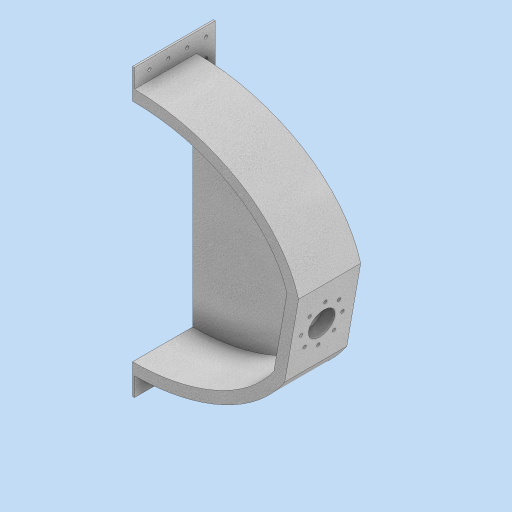
# Autodesk Inventor part: eggshellCorePrinted
Saved by Autodesk Inventor 2023 (Build 270158000, 158)
## iProperties
Created: 2026-03-19
Part Number: eggshellCorePrinted
Material: GFRC
Document SubType Name: Modeling
Designer: Nathann
Density: 1.7 g/cm^3
Appearance: Flat - Polished Gray
Mass: 7308.18 g
Surface Area: 8699.88 cm^2
Volume: 7308.18 cm^3
Author: Nathann
Autodesk Inventor part; units mm, degrees
ref_plane "YZ Plane" through (0, 0, 0) normal (1, 0, 0) x (0, 1, 0)
ref_plane "XZ Plane" through (0, 0, 0) normal (0, 1, 0) x (-1, 0, 0)
ref_plane "XY Plane" through (0, 0, 0) normal (0, 0, 1) x (1, 0, 0)
sketch "Sketch1" plane through (0, 0, 0) normal (0, 0, 1) x (1, 0, 0)
  ellipse E0 centre (0, 0) end of major axis (0, 330) minor radius 450 (0, -330) -> (0, 330) ccw
  ellipse E1 centre (0, 0) end of major axis (420, 0) minor radius 300 (0, -300) -> (0, 300) ccw
  line L0 (0, 300) -> (0, 330)
  line L1 (0, -300) -> (0, -330)
  line L2 (420, 0) -> (450, 0)
  dimension "d0" = 420
  dimension "d1" = 450
  dimension "d2" = 300
  dimension "d3" = 330
  constraints: 6 end point, 2 coincident, 2 point on line, 1 horizontal, 10 other
extrude "Extrusion1" add sketch "Sketch1" along normal blind 160
sketch "Sketch3" plane through (0, 0, 0) normal (0, 0, -1) x (-1, 0, 0)
  ellipse E0 centre (0, 0) end of major axis (420, 0) minor radius 300 (0, 300) -> (0, -300) ccw projected
  line L0 (-410.6033, 63.104) -> (-375.8737, -133.8576)
  line L1 (-375.8737, -133.8576) -> (-428.5073, -143.1383)
  line L2 (-428.5073, -143.1383) -> (-456.291, 14.4309)
  line L3 (0, 300) -> (0, -300) projected
  ellipse E1 centre (0, 0) end of major axis (450, 0) minor radius 330 (0, 330) -> (0, -330) ccw projected
  line L4 (-456.291, 14.4309) -> (-439.6592, 70.3382)
  line L5 (-428.5073, -143.1383) -> (-336.4493, -219.1451)
  line L6 (-336.4493, -219.1451) -> (-375.8737, -133.8576)
  line L7 (-410.6033, 63.104) -> (-439.6592, 70.3382)
  line L8 (-393.2385, -35.3768) -> (260.9914, 90.2506)
  line L9 (260.9914, 90.2506) -> (260.9914, 44.7879)
  line L10 (260.9914, 44.7879) -> (0, 40.1342)
  dimension "d8" = 200
  dimension "d9" = 10
  dimension "d12" = 45.4627
  dimension "d13" = 160
  constraints: 20 end point, 2 perpendicular, 2 point on line, 1 midpoint, 1 vertical, 9 other
  measures "d8" distance of L0.start L0.end
  measures "d9" angle of L3 L0
  measures "d12" distance of L8.end L9.end
  measures "d13" distance of L1.end L2.end
extrude "Extrusion2" add sketch "Sketch3" against normal blind 160 contours L0 E0
ref_plane "Work Plane2" through (0, 0, 0) normal (0, 0, -1) x (-1, 0, 0)
sketch "Sketch8" plane through (0, 0, 0) normal (0, 0, -1) x (-1, 0, 0)
  ellipse E0 centre (0, 0) end of major axis (450, 0) minor radius 330 (0, 330) -> (0, -330) ccw projected
  line L0 (0, -300) -> (0, -330) projected
  ellipse E1 centre (0, 0) end of major axis (420, 0) minor radius 300 (-375.8737, -133.8576) -> (0, -300) ccw projected
  line L1 (-375.8737, -133.8576) -> (-410.6033, 63.104) projected
  ellipse E2 centre (0, 0) end of major axis (420, 0) minor radius 300 (0, 300) -> (-410.6033, 63.104) ccw projected
  line L2 (0, 330) -> (0, 300) projected
  ellipse E3 centre (0, 0) end of major axis (420, 0) minor radius 300 (-375.8737, -133.8576) -> (0, -300) ccw projected
  line L3 (0, -300) -> (0, 300)
  point P0 (0, -300)
  constraints: 2 end point, 1 vertical, 5 other
extrude "Extrusion7" add sketch "Sketch8" along normal blind 5
ref_plane "Work Plane3" through (405.4179, -139.067, 0) normal (-0.9848078, 0.1736482, 0) x (0, 0, 1)
sketch "Sketch9" plane through (405.4179, -139.067, 0) normal (-0.9848078, 0.1736482, 0) x (0, 0, 1)
  line L0 (-87.5266, 298.4814) -> (215.3081, 298.4814)
  line L1 (215.3081, 298.4814) -> (215.3081, -153.555)
  line L2 (215.3081, -153.555) -> (-87.5266, -153.555)
  line L3 (-87.5266, -153.555) -> (-87.5266, 298.4814)
  point P0 (0, 66.5542)
  constraints: 8 end point, 2 parallel, 1 horizontal, 1 perpendicular
extrude "Extrusion8" cut sketch "Sketch9" against normal blind 60
sketch "Sketch10" plane through (0, 300, 160) normal (-1, 0, 0) x (0, 0, 1)
  line L0 (-160, -600) -> (0, -600) projected
  line L1 (0, -600) -> (-215, -600)
  line L2 (-215, -600) -> (-215, -680)
  line L3 (-215, -680) -> (0, -680)
  line L4 (0, -680) -> (0, -600)
  line L5 (-215, -600) -> (-165, -600)
  line L6 (-165, -600) -> (-165, 0)
  line L7 (-165, 80) -> (-215, 80)
  line L8 (-215, 80) -> (-215, -600)
  line L9 (0, 30) -> (0, 0) projected
  line L10 (-165, 80) -> (0, 80)
  line L11 (0, 80) -> (0, 30)
  line L12 (-165, 30) -> (-165, 80)
  line L13 (-165, -630) -> (-165, 30) projected
  circle A0 centre (-190, 55) radius 4.5
  circle A1 centre (-140, 55) radius 4.5
  circle A2 centre (-90, 55) radius 4.5
  circle A3 centre (-40, 55) radius 4.5
  circle A4 centre (-190, 5) radius 4.5
  circle A5 centre (-190, -45) radius 4.5
  circle A6 centre (-190, -95) radius 4.5
  circle A7 centre (-190, -145) radius 4.5
  circle A8 centre (-190, -195) radius 4.5
  circle A9 centre (-190, -245) radius 4.5
  line L14 (-165, -300) -> (-190, -300)
  line L15 (-165, 0) -> (-165, -600)
  circle A10 centre (-140, -655) radius 4.5
  circle A11 centre (-90, -655) radius 4.5
  circle A12 centre (-40, -655) radius 4.5
  circle A13 centre (-190, -605) radius 4.5
  circle A14 centre (-190, -555) radius 4.5
  circle A15 centre (-190, -505) radius 4.5
  circle A16 centre (-190, -455) radius 4.5
  circle A17 centre (-190, -405) radius 4.5
  circle A18 centre (-190, -355) radius 4.5
  circle A19 centre (-190, -655) radius 4.5
  line L16 (-160, 0) -> (0, 0) projected
  line L17 (0, 30) -> (0, 0)
  line L18 (0, 0) -> (-165, 0)
  point P0 (-160, -300)
  point P1 (0, -630)
  point P2 (-165, -680)
  point P3 (-165, -600)
  point P4 (-165, -600)
  point P5 (-215, -640)
  dimension "d38" = 50
  dimension "d40" = 9
  dimension "d41" = 25
  dimension "d42" = 25
  dimension "d45" = 50
  dimension "d52" = 50
  dimension "d57" = 9
  dimension "d73" = 50
  constraints: 30 end point, 20 centre point, 12 symmetric about line, 5 horizontal, 5 parallel, 3 perpendicular, 2 midpoint, 2 vertical, 1 coincident, 1 collinear, 27 other
  measures "d38" distance between parallel lines of L13 L2
  measures "d40" diameter of A0
  measures "d41" distance from line of L7 A0.centre
  measures "d42" distance from line of L8 A0.centre
  measures "d45" distance of A0.centre A1.centre
  measures "d52" distance of A0.centre A4.centre
  measures "d57" diameter of A19
  measures "d73" distance from line of point (-215, -640) L15
extrude "Extrusion9" add sketch "Sketch10" against normal blind 5
sketch "Sketch11" plane through (405.4179, -139.067, 0) normal (0.9848078, -0.1736482, 0) x (0, 0, -1)
  circle A0 centre (-80, 100.4954) radius 35
  line L0 (-160, -5.7359) -> (-160, 206.7266) projected
  line L1 (5, -5.7359) -> (-160, -5.7359) projected
  line L2 (-160, 206.7266) -> (5, 206.7266) projected
  circle A1 centre (-80, 155.4954) radius 4.5
  circle A2 centre (-118.8909, 139.3862) radius 4.5
  circle A3 centre (-135, 100.4954) radius 4.5
  circle A4 centre (-118.8909, 61.6045) radius 4.5
  circle A5 centre (-80, 45.4954) radius 4.5
  circle A6 centre (-41.1091, 61.6045) radius 4.5
  circle A7 centre (-25, 100.4954) radius 4.5
  circle A8 centre (-41.1091, 139.3862) radius 4.5
  point P0 (0, 66.5542)
  dimension "d60" = 70
  dimension "d61" = 80
  dimension "d62" = 106.2313
  dimension "d63" = 106.2313
  dimension "d64" = 212.4625
  dimension "d65" = 9
  dimension "d66" = 55
  dimension "d69" = 360
  constraints: 9 centre point, 17 other
  measures "d60" diameter of A0
  measures "d61" distance from line of L0 A0.centre
  measures "d62" distance from line of L1 A0.centre
  measures "d63" distance from line of L2 A0.centre
  measures "d64" distance between parallel lines of L1 L2
  measures "d65" diameter of A1
  measures "d66" distance of A0.centre A1.centre
extrude "Extrusion10" cut sketch "Sketch11" against normal blind 300
equation "\"d62\" = 0.5 * d64"
body "Solid1"
